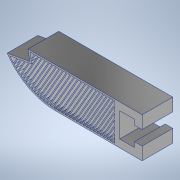
# Autodesk Inventor part: Finray_9_Kerbe_10deg
Saved by Autodesk Inventor 2022 (Build 260153000, 153)
## iProperties
Created: 2022-02-28
Part Number: Finray_9_Kerbe_10deg
Material: Generic
Document SubType Name: Modeling
Designer: richa
Density: 1 g/cm^3
Appearance: Aluminum - Flat
Author: richa
Autodesk Inventor part; units mm, degrees
ref_plane "YZ Plane" through (0, 0, 0) normal (1, 0, 0) x (0, 1, 0)
ref_plane "XZ Plane" through (0, 0, 0) normal (0, 1, 0) x (-1, 0, 0)
ref_plane "XY Plane" through (0, 0, 0) normal (0, 0, 1) x (1, 0, 0)
sketch "Sketch5" plane through (0, 0, 0) normal (0, 0, 1) x (1, 0, 0)
  line L0 (52.8, -15.6) -> (52.8, -10.6)
  line L1 (52.8, -10.6) -> (49.8, -10.6)
  line L2 (49.8, -10.6) -> (49.8, -12.6)
  line L3 (44, -12.6) -> (44, -3)
  line L4 (49.8, -3) -> (49.8, -5)
  line L5 (49.8, -5) -> (52.8, -5)
  line L6 (52.8, -5) -> (52.8, 0)
  line L7 (52.8, 0) -> (7.8, 0)
  line L8 (44, -3) -> (49.8, -3)
  line L9 (44, -12.6) -> (49.8, -12.6)
  line L10 (52.8, -15.6) -> (7.8, -15.6)
  line L11 (7.8, -15.6) -> (0, -15.6)
  line L12 (0, -15.6) -> (0, 0)
  line L13 (0, 0) -> (7.8, 0)
  point P0 (7.8, 0)
  dimension "d41" = 5.8
  dimension "d48" = 44
  dimension "d50" = 3
  dimension "d63" = 45
  dimension "d71" = 0
  dimension "d87" = 5.6
  dimension "d88" = 9.6
  dimension "d97" = 15.6
  constraints: 28 end point, 8 perpendicular, 4 collinear, 3 parallel, 2 horizontal, 1 vertical
  measures "d41" distance between parallel lines of L2 L3
  measures "d48" distance from line of L3 L12.end
  measures "d50" distance of L4.end L5.end
  measures "d63" distance of L0.start L10.end
  measures "d71" distance from line of L12.end L7
  measures "d87" distance from line of L0.end L5
  measures "d88" distance of L3.start L3.end
  measures "d97" distance of L11.end L12.end
extrude "Extrusion2" add sketch "Sketch5" along normal blind 12
sketch "Sketch8" plane through (0, 0, 0) normal (0, 0, -1) x (-1, 0, 0)
  line L0 (-8.1687, 0) -> (-8.8633, -3.9392)
  line L1 (-7.8, 0) -> (-1.143, 0) construction
  line L2 (0, -5.5021) -> (-8.8633, -3.9392)
  line L3 (-7.8, 0) -> (-8.1687, 0)
  line L4 (0, 0) -> (0, -15.6) projected
  line L5 (-52.8, 0) -> (0, 0) projected
  line L6 (-7.8, 0) -> (0, 0)
  line L7 (0, 0) -> (0, -5.5021)
  dimension "d80" = 100
  dimension "d95" = 4
  dimension "d96" = 9
  constraints: 12 end point, 2 collinear, 2 perpendicular, 1 horizontal, 1 point on line
  measures "d80" angle of L0 L1
  measures "d95" distance of L0.start L0.end
  measures "d96" distance of L2.start L0.end
extrude "Extrusion5" cut sketch "Sketch8" against normal through all
fillet "Fillet2" radius 23 1 edges at (0, -15.6, 6)
shell "Shell1" thickness 0.62 removed faces 1 at (23.9679, -7.5131, 12)
sketch "Sketch13" plane through (0, 0, 12) normal (0, 0, 1) x (1, 0, 0)
  line L0 (19.0404, -15.6) -> (52.8, -15.6) projected
  line L1 (42.0526, -15.6) -> (42.0526, 0)
  line L2 (52.8, 0) -> (8.1687, 0) projected
  line L3 (52.8, 0) -> (8.1687, 0) projected
  line L4 (52.8, -5) -> (52.8, 0) projected
  line L5 (49.8, -5) -> (52.8, -5) projected
  line L6 (49.8, -3) -> (49.8, -5) projected
  line L7 (44, -3) -> (49.8, -3) projected
  line L8 (44, -12.6) -> (44, -3) projected
  line L9 (49.8, -12.6) -> (44, -12.6) projected
  line L10 (49.8, -10.6) -> (49.8, -12.6) projected
  line L11 (52.8, -10.6) -> (49.8, -10.6) projected
  line L12 (52.8, -15.6) -> (52.8, -10.6) projected
  line L13 (42.0526, 0) -> (52.8, 0)
  line L14 (52.8, -5) -> (52.8, 0) projected
  line L15 (52.8, -5) -> (52.8, 0)
  line L16 (52.8, 0) -> (52.8, -5)
  line L17 (44, -12.6) -> (44, -3) projected
  line L18 (44, -3) -> (44, -12.6)
  line L19 (49.8, -12.6) -> (44, -12.6) projected
  line L20 (44, -12.6) -> (49.8, -12.6)
  line L21 (43.38, -13.22) -> (50.42, -13.22) projected
  line L22 (52.8, -10.6) -> (52.8, -15.6)
  line L23 (52.8, -15.6) -> (42.0526, -15.6)
  line L24 (44, -3) -> (49.8, -3) projected
  line L25 (44, -3) -> (49.8, -3)
  line L26 (49.8, -3) -> (49.8, -5)
  line L27 (49.8, -5) -> (52.8, -5)
  line L28 (52.8, -10.6) -> (49.8, -10.6)
  line L29 (49.8, -10.6) -> (49.8, -12.6)
  point P0 (0, 0)
  dimension "d102" = 10.7474
  constraints: 26 end point, 10 collinear, 2 point on line, 2 vertical, 1 parallel
  measures "d102" distance between parallel lines of L4 L1
extrude "Extrusion7" add sketch "Sketch13" against normal blind 12
sketch "Sketch14" plane through (8.9076, -0.62, 0.62) normal (0, 0, 1) x (1, 0, 0)
  line L0 (33.145, -14.36) -> (33.145, 0) projected
  line L1 (33.145, 0) -> (0, 0) projected
  line L2 (0.6739, -3.8221) -> (0, 0) projected
  line L3 (-7.835, -5.3225) -> (0.6739, -3.8221) projected
  arc A0 (-7.835, -5.3225) -> (10.1328, -14.36) centre (10.1328, 8.02) ccw projected
  line L4 (10.1328, -14.36) -> (33.145, -14.36) projected
  point P0 (-8.9076, 0.62)
extrude "Extrusion8" cut sketch "Sketch14" against normal blind 12
sketch "Sketch15" plane through (0, 0, 12) normal (0, 0, 1) x (1, 0, 0)
  line L0 (42.0526, -0.62) -> (8.9076, -0.62) construction
  line L1 (19.0404, -14.98) -> (42.0526, -14.98) projected
  line L2 (45.8641, -0.62) -> (37.5734, -14.98)
  line L3 (37.1346, -14.98) -> (45.4253, -0.62)
  line L4 (41.8778, -0.62) -> (33.587, -14.98)
  line L5 (33.1482, -14.98) -> (41.439, -0.62)
  line L6 (37.8914, -0.62) -> (29.6006, -14.98)
  line L7 (29.1619, -14.98) -> (37.4526, -0.62)
  line L8 (33.7674, -0.62) -> (25.4766, -14.98)
  line L9 (25.0643, -14.98) -> (33.355, -0.62)
  line L10 (29.3944, -0.62) -> (21.1037, -14.98)
  line L11 (20.6649, -14.98) -> (28.9556, -0.62)
  line L12 (24.995, -0.62) -> (16.5053, -15.3245)
  line L13 (16.5053, -15.3245) -> (16.1071, -15.2543)
  line L14 (16.1071, -15.2543) -> (24.5562, -0.62)
  line L15 (20.7333, -0.62) -> (12.6135, -14.6838)
  line L16 (16.6092, -0.62) -> (9.2293, -13.4024)
  line L17 (8.886, -13.2371) -> (16.1704, -0.62)
  arc A0 (1.0726, -5.9425) -> (19.0404, -14.98) centre (19.0404, 7.4) ccw projected
  line L18 (42.0526, -0.62) -> (42.0526, -14.98) projected
  line L19 (1.0726, -5.9425) -> (9.5815, -4.4421) projected
  arc A1 (0, -5.5021) -> (19.0404, -15.6) centre (19.0404, 7.4) ccw projected
  line L20 (7.8435, -0.62) -> (3.2927, -8.5021)
  line L21 (3.5737, -8.7755) -> (8.2822, -0.62)
  line L22 (11.9675, -0.62) -> (6.0686, -10.8372)
  line L23 (6.3813, -11.0556) -> (12.4063, -0.62)
  line L24 (42.0526, -14.98) -> (19.0404, -14.98) projected
  line L25 (39.7921, -14.98) -> (40.1212, -15.17)
  line L26 (40.1212, -15.17) -> (48.5217, -0.62)
  line L27 (48.5217, -0.62) -> (48.0829, -0.62)
  line L28 (48.0829, -0.62) -> (39.7921, -14.98)
  line L29 (8.9076, -0.62) -> (42.0526, -0.62) projected
  line L30 (44.0965, -0.62) -> (44.5353, -0.62)
  line L31 (44.5353, -0.62) -> (36.2446, -14.98)
  line L32 (36.2446, -14.98) -> (35.8058, -14.98)
  line L33 (35.8058, -14.98) -> (44.0965, -0.62)
  line L34 (40.1102, -0.62) -> (40.549, -0.62)
  line L35 (40.549, -0.62) -> (32.2582, -14.98)
  line L36 (32.2582, -14.98) -> (31.8194, -14.98)
  line L37 (31.8194, -14.98) -> (40.1102, -0.62)
  line L38 (36.1238, -0.62) -> (36.5626, -0.62)
  line L39 (36.5626, -0.62) -> (28.2719, -14.98)
  line L40 (28.2719, -14.98) -> (27.8331, -14.98)
  line L41 (27.8331, -14.98) -> (36.1238, -0.62)
  line L42 (31.8886, -0.62) -> (32.3273, -0.62)
  line L43 (32.3273, -0.62) -> (24.0366, -14.98)
  line L44 (24.0366, -14.98) -> (23.5978, -14.98)
  line L45 (23.5978, -14.98) -> (31.8886, -0.62)
  line L46 (27.4891, -0.62) -> (27.9279, -0.62)
  line L47 (27.9279, -0.62) -> (19.6372, -14.98)
  line L48 (19.6372, -14.98) -> (19.1984, -14.98)
  line L49 (19.1984, -14.98) -> (27.4891, -0.62)
  line L50 (23.0897, -0.62) -> (23.5285, -0.62)
  line L51 (23.5285, -0.62) -> (15.409, -14.6834)
  line L52 (15.409, -14.6834) -> (14.9702, -14.6834)
  line L53 (14.9702, -14.6834) -> (23.0897, -0.62)
  line L54 (18.9657, -0.62) -> (19.4045, -0.62)
  line L55 (19.4045, -0.62) -> (11.8072, -13.7789)
  line L56 (11.8072, -13.7789) -> (11.3684, -13.7789)
  line L57 (11.3684, -13.7789) -> (18.9657, -0.62)
  line L58 (14.704, -0.62) -> (15.1428, -0.62)
  line L59 (15.1428, -0.62) -> (8.4044, -12.2911)
  line L60 (8.4044, -12.2911) -> (7.9656, -12.2911)
  line L61 (7.9656, -12.2911) -> (14.704, -0.62)
  line L62 (6.9535, -0.62) -> (2.7339, -7.9285)
  line L63 (2.4639, -7.6361) -> (6.5147, -0.62)
  line L64 (8.7902, -4.5817) -> (8.3514, -4.5817)
  line L65 (10.6387, -0.62) -> (5.1417, -10.1411)
  line L66 (5.4444, -10.3768) -> (11.0775, -0.62)
  line L67 (46.7541, -0.62) -> (47.1929, -0.62)
  line L68 (47.1929, -0.62) -> (38.9021, -14.98)
  line L69 (38.9021, -14.98) -> (38.4634, -14.98)
  line L70 (38.4634, -14.98) -> (46.7541, -0.62)
  line L71 (42.7678, -0.62) -> (43.2065, -0.62)
  line L72 (43.2065, -0.62) -> (34.9158, -14.98)
  line L73 (34.9158, -14.98) -> (34.477, -14.98)
  line L74 (34.477, -14.98) -> (42.7678, -0.62)
  line L75 (38.7814, -0.62) -> (39.2202, -0.62)
  line L76 (39.2202, -0.62) -> (30.9294, -14.98)
  line L77 (30.9294, -14.98) -> (30.4906, -14.98)
  line L78 (30.4906, -14.98) -> (38.7814, -0.62)
  line L79 (34.795, -0.62) -> (35.2338, -0.62)
  line L80 (35.2338, -0.62) -> (26.9431, -14.98)
  line L81 (26.9431, -14.98) -> (26.5043, -14.98)
  line L82 (26.5043, -14.98) -> (34.795, -0.62)
  line L83 (30.4221, -0.62) -> (30.8609, -0.62)
  line L84 (30.8609, -0.62) -> (22.5701, -14.98)
  line L85 (22.5701, -14.98) -> (22.1313, -14.98)
  line L86 (22.1313, -14.98) -> (30.4221, -0.62)
  line L87 (26.0227, -0.62) -> (26.4615, -0.62)
  line L88 (26.4615, -0.62) -> (18.1707, -14.98)
  line L89 (18.1707, -14.98) -> (17.7319, -14.98)
  line L90 (17.7319, -14.98) -> (26.0227, -0.62)
  line L91 (21.6233, -0.62) -> (22.0621, -0.62)
  line L92 (22.0621, -0.62) -> (14.0912, -14.4259)
  line L93 (14.0912, -14.4259) -> (13.6524, -14.4259)
  line L94 (13.6524, -14.4259) -> (21.6233, -0.62)
  line L95 (17.4992, -0.62) -> (17.938, -0.62)
  line L96 (17.938, -0.62) -> (10.6011, -13.3278)
  line L97 (10.6011, -13.3278) -> (10.1624, -13.3278)
  line L98 (10.1624, -13.3278) -> (17.4992, -0.62)
  line L99 (7.1575, -4.8696) -> (6.7188, -4.8696)
  line L100 (9.1722, -0.62) -> (4.1543, -9.3113)
  line L101 (4.4458, -9.5665) -> (9.611, -0.62)
  line L102 (13.6763, -0.62) -> (13.2963, -0.62)
  line L103 (13.2963, -0.62) -> (7.0255, -11.4814)
  line L104 (7.3046, -11.6561) -> (13.6763, -0.62)
  line L105 (8.9076, -0.62) -> (-0.0004, -0.62) construction
  line L106 (45.4253, -0.62) -> (45.8641, -0.62)
  line L107 (12.5577, -14.0205) -> (20.2945, -0.62)
  point P0 (0, 0)
  point P1 (38.1346, -13.248)
  point P2 (41.2007, -1.0328)
  point P3 (33.6831, -14.8136)
  point P4 (41.5989, -1.103)
  point P5 (33.2608, -14.7849)
  point P6 (37.2598, -0.9539)
  point P7 (29.8469, -14.5535)
  point P8 (29.2745, -14.7849)
  point P9 (32.0327, -2.9103)
  point P10 (32.407, -2.9762)
  point P11 (28.0398, -2.2062)
  point P12 (28.4381, -2.2764)
  point P13 (24.0469, -1.5021)
  point P14 (24.4452, -1.5724)
  point P15 (20.0562, -1.0328)
  point P16 (20.4544, -1.103)
  point P17 (15.7017, -1.4319)
  point P18 (16.0999, -1.5021)
  point P19 (5.6782, -5.1304)
  point P20 (5.5025, -4.6747)
  point P21 (6.3658, -10.3225)
  point P22 (6.7278, -10.4554)
  point P23 (37.1346, -14.98)
  point P24 (33.1482, -14.98)
  point P25 (33.587, -14.98)
  point P26 (29.4219, -14.98)
  point P27 (29.6006, -14.98)
  point P28 (21.1037, -14.98)
  point P29 (19.6462, -14.98)
  point P30 (20.0321, -14.98)
  point P31 (9.1967, -12.6989)
  point P32 (9.5404, -12.8636)
  point P33 (3.7102, -5.4774)
  point P34 (3.7963, -6.0884)
  point P35 (2.5646, -7.4617)
  point P36 (5.5087, -9.5055)
  point P37 (5.8581, -9.6603)
  point P38 (39.7921, -14.98)
  point P39 (40.2309, -14.98)
  point P40 (35.8058, -14.98)
  point P41 (36.2446, -14.98)
  point P42 (41.7312, -0.62)
  point P43 (40.1102, -0.62)
  point P44 (31.8194, -14.98)
  point P45 (32.2582, -14.98)
  point P46 (40.549, -0.62)
  point P47 (36.1238, -0.62)
  point P48 (27.8331, -14.98)
  point P49 (28.2719, -14.98)
  point P50 (36.5626, -0.62)
  point P51 (31.8886, -0.62)
  point P52 (23.5978, -14.98)
  point P53 (24.0366, -14.98)
  point P54 (32.3273, -0.62)
  point P55 (27.4891, -0.62)
  point P56 (19.1984, -14.98)
  point P57 (19.6372, -14.98)
  point P58 (27.9279, -0.62)
  point P59 (23.5285, -0.62)
  point P60 (19.4045, -0.62)
  point P61 (15.1428, -0.62)
  point P62 (4.9424, -7.9464)
  point P63 (5.3185, -8.0549)
  point P64 (7.0923, -11.3656)
  point P65 (7.4723, -11.3656)
  point P66 (38.4634, -14.98)
  point P67 (38.9021, -14.98)
  point P68 (41.9433, -0.62)
  point P69 (34.477, -14.98)
  point P70 (34.9158, -14.98)
  point P71 (40.4024, -0.62)
  point P72 (30.4906, -14.98)
  point P73 (30.9294, -14.98)
  point P74 (39.2202, -0.62)
  point P75 (26.5043, -14.98)
  point P76 (26.9431, -14.98)
  point P77 (35.2338, -0.62)
  point P78 (22.1313, -14.98)
  point P79 (22.5701, -14.98)
  point P80 (30.8609, -0.62)
  point P81 (19.6871, -14.98)
  point P82 (19.1528, -14.98)
  point P83 (26.4615, -0.62)
  point P84 (22.0621, -0.62)
  point P85 (17.938, -0.62)
  point P86 (13.2963, -0.62)
  point P87 (4.1988, -5.3913)
  point P88 (5.1896, -5.2166)
  point P89 (6.669, -4.9557)
  point P90 (8.3017, -4.6678)
  point P91 (9.0662, -4.533)
  point P92 (9.3039, -4.4911)
  point P93 (12.933, -14.1305)
  point P94 (12.4063, -0.62)
  point P95 (11.9675, -0.62)
  point P96 (11.0775, -0.62)
  point P97 (10.6387, -0.62)
  point P98 (17.1982, -15.5261)
  point P99 (17.5923, -15.5544)
  point P100 (24.5562, -0.62)
  point P101 (16.3586, -14.8187)
  point P102 (16.7709, -14.8646)
  dimension "d105" = 0.38
  dimension "d107" = 0.38
  dimension "d110" = 0.38
  dimension "d111" = 0.38
  dimension "d113" = 0.38
  dimension "d129" = 0.38
  dimension "d131" = 0.38
  dimension "d132" = 0.38
  dimension "d133" = 0.38
  dimension "d134" = 0.38
  dimension "d135" = 0.38
  dimension "d136" = 0.38
  dimension "d137" = 0.38
  dimension "d138" = 0.38
  dimension "d139" = 0.38
  dimension "d151" = 0.38
  dimension "d157" = 0.38
  dimension "d161" = 0.38
  dimension "d163" = 0.38
  dimension "d168" = 0.89
  dimension "d169" = 0.38
  dimension "d170" = 0.89
  dimension "d171" = 0.89
  dimension "d172" = 0.38
  dimension "d173" = 0.89
  dimension "d175" = 0.38
  dimension "d176" = 0.89
  dimension "d178" = 0.38
  dimension "d179" = 0.89
  dimension "d182" = 0.89
  dimension "d184" = 0.89
  dimension "d185" = 120
  dimension "d186" = 120
  dimension "d187" = 120
  dimension "d189" = 0.89
  dimension "d193" = 0.89
  dimension "d194" = 0.89
  dimension "d195" = 0.89
  dimension "d196" = 0.89
  dimension "d197" = 0.89
  dimension "d200" = 0.38
  dimension "d201" = 120
  dimension "d202" = 0.89
  dimension "d205" = 0.89
  dimension "d206" = 0.89
  dimension "d207" = 0.89
  dimension "d209" = 0.89
  dimension "d210" = 0.38
  dimension "d211" = 0.38
  dimension "d213" = 0.89
  dimension "d214" = 0.38
  dimension "d215" = 0.38
  dimension "d216" = 0.38
  dimension "d217" = 0.89
  dimension "d218" = 0.89
  dimension "d221" = 0.89
  dimension "d222" = 0.89
  dimension "d223" = 0.89
  dimension "d224" = 0.38
  dimension "d225" = 0.89
  dimension "d226" = 0.89
  dimension "d227" = 0.89
  dimension "d228" = 0.89
  dimension "d229" = 0.89
  constraints: 202 end point, 57 parallel, 45 point on line, 20 horizontal, 3 point on circle, 1 collinear, 1 perpendicular, 83 other
  measures "d105" distance between parallel lines of L2 L3
  measures "d107" distance between parallel lines of L4 L5
  measures "d110" distance between parallel lines of L10 L11
  measures "d111" distance between parallel lines of L12 L14
  measures "d113" distance between parallel lines of L16 L17
  measures "d129" distance between parallel lines of L26 L28
  measures "d131" distance between parallel lines of L31 L33
  measures "d132" distance between parallel lines of L35 L37
  measures "d133" distance between parallel lines of L39 L41
  measures "d134" distance between parallel lines of L43 L45
  measures "d135" distance between parallel lines of L47 L49
  measures "d136" distance between parallel lines of L51 L53
  measures "d137" distance between parallel lines of L55 L57
  measures "d138" distance between parallel lines of L59 L61
  measures "d139" distance between parallel lines of L66 L65
  measures "d151" distance between parallel lines of L68 L70
  measures "d157" distance between parallel lines of L72 L74
  measures "d161" distance between parallel lines of L76 L78
  measures "d163" distance between parallel lines of L80 L82
  measures "d168" distance between parallel lines of L11 L47
  measures "d169" distance between parallel lines of L88 L90
  measures "d170" distance between parallel lines of L49 L88
  measures "d171" distance between parallel lines of L14 L51
  measures "d172" distance between parallel lines of L92 L94
  measures "d173" distance between parallel lines of L53 L92
  measures "d175" distance between parallel lines of L96 L98
  measures "d176" distance between parallel lines of L57 L96
  measures "d178" distance of L102.start L102.end
  measures "d179" distance between parallel lines of L61 L104
  measures "d182" distance between parallel lines of L65 L101
  measures "d184" distance between parallel lines of L17 L59
  measures "d185" angle to the sketch x axis of L26
  measures "d186" angle of L0 L31
  measures "d187" angle of L0 L2
  measures "d189" distance of L34.start L75.end
  measures "d193" distance between parallel lines of L82 L8
  measures "d194" distance between parallel lines of L9 L43
  measures "d195" distance between parallel lines of L45 L84
  measures "d196" distance between parallel lines of L86 L10
  measures "d197" distance between parallel lines of L90 L12
  measures "d200" distance between parallel lines of L84 L86
  measures "d201" angle of L0 L92
  measures "d202" distance of L102.end L23.end
  measures "d205" distance of L30.start L71.end
  measures "d206" distance of L3.end L30.end
  measures "d207" distance of L67.start L2.start
  measures "d209" distance of L27.end L67.end
  measures "d210" distance between parallel lines of L23 L22
  measures "d211" distance between parallel lines of L15 L107
  measures "d213" distance of L22.start L66.end
  measures "d214" distance between parallel lines of L101 L100
  measures "d215" distance between parallel lines of L20 L21
  measures "d216" distance between parallel lines of L63 L62
  measures "d217" distance of L100.start L21.end
  measures "d218" distance of L20.start L62.start
  measures "d221" distance of L95.start L16.start
  measures "d222" distance of L107.end L54.end
  measures "d223" distance of L91.start L15.start
  measures "d224" distance between parallel lines of L6 L7
  measures "d225" distance of L4.start L71.start
  measures "d226" distance of L34.end L5.end
  measures "d227" distance of L7.end L38.end
  measures "d228" distance of L75.start L6.start
  measures "d229" distance of L38.start L79.end
extrude "Extrusion9" add sketch "Sketch15" against normal blind 12 contours L49 L29 L47 L1 | L88 L89 L90 A0 | A0 L90 L29 L88 | L11 L29 L10 L1 | A0 L14 L29 L12 | L86 L29 L84 L1 | L52 L53 A0 | A0 L53 L29 L51 | L45 L29 L43 L1 | L93 L94 A0 | A0 L94 L29 L92 | L9 L29 L8 L1 | A0 L107 L29 L15 | L82 L29 L80 L1 | L56 L57 A0 | A0 L57 L29 L55 | A0 L17 L29 L16 | L41 L29 L39 L1 | L98 L29 L96 A0 | A0 L97 L98 | L60 L61 A0 | A0 L61 L29 L59 | L7 L29 L6 L1 | A0 L103 L29 L104 | L78 L29 L76 L1 | A0 L22 L29 L23 | L37 L29 L35 L1 | A0 L65 L19 L66 | L5 L29 L4 L1 | L66 L64 L65 L29 | L19 L65 L64 | A0 L100 L19 L101 | L74 L18 L72 L1 | L19 L100 L99 | L74 L71 L72 L18 | A0 L20 L19 L21 | L33 L18 L31 L1 | L33 L30 L31 L18 | A0 L63 L19 L62 | L3 L18 L2 L1 | L3 L106 L2 L18 | L70 L18 L68 L1 | L70 L67 L68 L18 | L28 L18 L26 L1 | L28 L27 L26 L18
sketch "Sketch16" plane through (0, 0, 12) normal (0, 0, 1) x (1, 0, 0)
  arc A0 (0, -5.5021) -> (19.0404, -15.6) centre (19.0404, 7.4) ccw projected
  line L0 (9.3126, -2.9169) -> (8.9076, -0.62) projected
  line L1 (8.1687, 0) -> (8.8303, -3.7523) projected
  line L2 (8.1687, 0) -> (8.8633, -3.9392)
  line L3 (52.8, 0) -> (8.1687, 0) projected
  line L4 (0, -5.5021) -> (8.1687, 0)
  line L5 (0, -5.5021) -> (8.8633, -3.9392)
  point P0 (0, 0)
  point P1 (9.5815, -4.4421)
  point P2 (9.3319, -3.0264)
  point P3 (8.8242, -3.7175)
  point P4 (9.4967, -3.9613)
  constraints: 6 end point, 1 collinear, 1 perpendicular
extrude "Extrusion10" cut sketch "Sketch16" against normal blind 12
sketch "Sketch17" plane through (0, 0, 12) normal (0, 0, 1) x (1, 0, 0)
  line L0 (49.8, -12.6) -> (44, -12.6) projected
  line L1 (49.8, -3) -> (49.8, -5) projected
  line L2 (44, -12.6) -> (49.8, -12.6)
  line L3 (49.8, -12.6) -> (49.8, -3)
  line L4 (49.8, -3) -> (44, -3)
  line L5 (44, -3) -> (44, -12.6)
  point P0 (0, 0)
  constraints: 8 end point, 2 parallel, 1 horizontal, 1 perpendicular
extrude "Extrusion11" cut sketch "Sketch17" against normal blind 12
equation "\"l1\" = 8"
equation "\"d1\" = 0.38"
body "Solid2"
